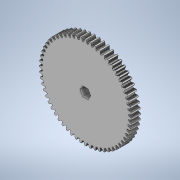
# Autodesk Inventor part: Engranajes_60
Saved by Autodesk Inventor 2022 (Build 260153000, 153)
## iProperties
Created: 2022-02-21
Part Number: Engranajes_60
Material: Generic
Document SubType Name: Modeling
Designer: katha
Density: 1 g/cm^3
Appearance: Default
Author: katha
Autodesk Inventor part; units mm, degrees
(part 1 of 6)
ref_plane "YZ Plane" through (0, 0, 0) normal (1, 0, 0) x (0, 1, 0)
ref_plane "XZ Plane" through (0, 0, 0) normal (0, 1, 0) x (-1, 0, 0)
ref_plane "XY Plane" through (0, 0, 0) normal (0, 0, 1) x (1, 0, 0)
sketch "Sketch1" plane through (0, 0, 0) normal (0, 0, 1) x (1, 0, 0)
  circle A0 centre (37.5, 0) radius 2
  circle A1 centre (0, 0) radius 2
  circle A2 centre (37.5, 0) radius 2
  circle A3 centre (0, 0) radius 2
  line L0 (30.5004, -4.5761) -> (30.5788, -4.4112)
  line L1 (30.5788, -4.4112) -> (30.6581, -4.2611)
  line L2 (30.6581, -4.2611) -> (30.7375, -4.1249)
  line L3 (30.7375, -4.1249) -> (30.8151, -4.0037)
  line L4 (30.8151, -4.0037) -> (30.8928, -3.8929)
  line L5 (30.8928, -3.8929) -> (30.9659, -3.7975)
  line L6 (30.9659, -3.7975) -> (31.0351, -3.7146)
  line L7 (31.0351, -3.7146) -> (31.0995, -3.6436)
  line L8 (31.0995, -3.6436) -> (31.1577, -3.5847)
  line L9 (31.1577, -3.5847) -> (31.2544, -3.498)
  line L10 (31.2544, -3.498) -> (31.3364, -3.4375)
  line L11 (31.3364, -3.4375) -> (31.3874, -3.4115)
  line L12 (31.3874, -3.4115) -> (31.4881, -3.3539)
  line L13 (31.4881, -3.3539) -> (31.5734, -3.2945)
  line L14 (31.5734, -3.2945) -> (31.6432, -3.2343)
  line L15 (31.6432, -3.2343) -> (31.6977, -3.1746)
  line L16 (31.6977, -3.1746) -> (31.7371, -3.1165)
  line L17 (31.7371, -3.1165) -> (31.7616, -3.0612)
  line L18 (31.7616, -3.0612) -> (31.7684, -3.035)
  line L19 (31.7684, -3.035) -> (31.7716, -3.0098)
  line L20 (31.7716, -3.0098) -> (31.7712, -2.986)
  line L21 (31.7712, -2.986) -> (31.7674, -2.9635)
  line L22 (31.7674, -2.9635) -> (31.7578, -2.9376)
  line L23 (31.7578, -2.9376) -> (31.6423, -2.7)
  line L24 (31.6423, -2.7) -> (31.6076, -2.6235)
  line L25 (31.6076, -2.6235) -> (31.5739, -2.5464)
  line L26 (31.5739, -2.5464) -> (31.4746, -2.3016)
  line L27 (31.4746, -2.3016) -> (31.4618, -2.2772)
  line L28 (31.4618, -2.2772) -> (31.4477, -2.2593)
  line L29 (31.4477, -2.2593) -> (31.4302, -2.2431)
  line L30 (31.4302, -2.2431) -> (31.4094, -2.2286)
  line L31 (31.4094, -2.2286) -> (31.3854, -2.2161)
  line L32 (31.3854, -2.2161) -> (31.3279, -2.1973)
  line L33 (31.3279, -2.1973) -> (31.2584, -2.1877)
  line L34 (31.2584, -2.1877) -> (31.1775, -2.1883)
  line L35 (31.1775, -2.1883) -> (31.0861, -2.1999)
  line L36 (31.0861, -2.1999) -> (30.9848, -2.2234)
  line L37 (30.9848, -2.2234) -> (30.8747, -2.2598)
  line L38 (30.8747, -2.2598) -> (30.8212, -2.2803)
  line L39 (30.8212, -2.2803) -> (30.7213, -2.3008)
  line L40 (30.7213, -2.3008) -> (30.5923, -2.3146)
  line L41 (30.5923, -2.3146) -> (30.5095, -2.3184)
  line L42 (30.5095, -2.3184) -> (30.4137, -2.3188)
  line L43 (30.4137, -2.3188) -> (30.3057, -2.3148)
  line L44 (30.3057, -2.3148) -> (30.186, -2.3053)
  line L45 (30.186, -2.3053) -> (30.0516, -2.2888)
  line L46 (30.0516, -2.2888) -> (29.9096, -2.2654)
  line L47 (29.9096, -2.2654) -> (29.7552, -2.2333)
  line L48 (29.7552, -2.2333) -> (29.5907, -2.1918)
  line L49 (29.5907, -2.1918) -> (29.4157, -2.1397)
  line L50 (29.4157, -2.1397) -> (29.2602, -2.0868)
  arc A4 (29.1238, -1.4451) -> (29.2602, -2.0868) centre (37.5, 0) ccw
  line L51 (29.1238, -1.4451) -> (29.2443, -1.3335)
  line L52 (29.2443, -1.3335) -> (29.383, -1.2147)
  line L53 (29.383, -1.2147) -> (29.5164, -1.1099)
  line L54 (29.5164, -1.1099) -> (29.6444, -1.0178)
  line L55 (29.6444, -1.0178) -> (29.7646, -0.9386)
  line L56 (29.7646, -0.9386) -> (29.8807, -0.8689)
  line L57 (29.8807, -0.8689) -> (29.9862, -0.8115)
  line L58 (29.9862, -0.8115) -> (30.0832, -0.7639)
  line L59 (30.0832, -0.7639) -> (30.1709, -0.7253)
  line L60 (30.1709, -0.7253) -> (30.248, -0.6951)
  line L61 (30.248, -0.6951) -> (30.3716, -0.6552)
  line L62 (30.3716, -0.6552) -> (30.4711, -0.6334)
  line L63 (30.4711, -0.6334) -> (30.5283, -0.6304)
  line L64 (30.5283, -0.6304) -> (30.6437, -0.6187)
  line L65 (30.6437, -0.6187) -> (30.7458, -0.5991)
  line L66 (30.7458, -0.5991) -> (30.8341, -0.5725)
  line L67 (30.8341, -0.5725) -> (30.9081, -0.5401)
  line L68 (30.9081, -0.5401) -> (30.9677, -0.5031)
  line L69 (30.9677, -0.5031) -> (31.0126, -0.4625)
  line L70 (31.0126, -0.4625) -> (31.0295, -0.4413)
  line L71 (31.0295, -0.4413) -> (31.0426, -0.4197)
  line L72 (31.0426, -0.4197) -> (31.052, -0.3977)
  line L73 (31.052, -0.3977) -> (31.0576, -0.3757)
  line L74 (31.0576, -0.3757) -> (31.0594, -0.3481)
  line L75 (31.0594, -0.3481) -> (31.0505, -0.0841)
  line L76 (31.0505, -0.0841) -> (31.05, 0)
  line L77 (31.05, 0) -> (31.0505, 0.0841)
  line L78 (31.0505, 0.0841) -> (31.0594, 0.3481)
  line L79 (31.0594, 0.3481) -> (31.0576, 0.3757)
  line L80 (31.0576, 0.3757) -> (31.052, 0.3977)
  line L81 (31.052, 0.3977) -> (31.0426, 0.4197)
  line L82 (31.0426, 0.4197) -> (31.0295, 0.4413)
  line L83 (31.0295, 0.4413) -> (31.0126, 0.4625)
  line L84 (31.0126, 0.4625) -> (30.9677, 0.5031)
  line L85 (30.9677, 0.5031) -> (30.9081, 0.5401)
  line L86 (30.9081, 0.5401) -> (30.8341, 0.5725)
  line L87 (30.8341, 0.5725) -> (30.7458, 0.5991)
  line L88 (30.7458, 0.5991) -> (30.6437, 0.6187)
  line L89 (30.6437, 0.6187) -> (30.5283, 0.6304)
  line L90 (30.5283, 0.6304) -> (30.4711, 0.6334)
  line L91 (30.4711, 0.6334) -> (30.3716, 0.6552)
  line L92 (30.3716, 0.6552) -> (30.248, 0.6951)
  line L93 (30.248, 0.6951) -> (30.1709, 0.7253)
  line L94 (30.1709, 0.7253) -> (30.0832, 0.7639)
  line L95 (30.0832, 0.7639) -> (29.9862, 0.8115)
  line L96 (29.9862, 0.8115) -> (29.8807, 0.8689)
  line L97 (29.8807, 0.8689) -> (29.7646, 0.9386)
  line L98 (29.7646, 0.9386) -> (29.6444, 1.0178)
  line L99 (29.6444, 1.0178) -> (29.5164, 1.1099)
  line L100 (29.5164, 1.1099) -> (29.383, 1.2147)
  line L101 (29.383, 1.2147) -> (29.2443, 1.3335)
  line L102 (29.2443, 1.3335) -> (29.1238, 1.4451)
  arc A5 (29.2602, 2.0868) -> (29.1238, 1.4451) centre (37.5, 0) ccw
  line L103 (29.2602, 2.0868) -> (29.4157, 2.1397)
  line L104 (29.4157, 2.1397) -> (29.5907, 2.1918)
  line L105 (29.5907, 2.1918) -> (29.7552, 2.2333)
  line L106 (29.7552, 2.2333) -> (29.9096, 2.2654)
  line L107 (29.9096, 2.2654) -> (30.0516, 2.2888)
  line L108 (30.0516, 2.2888) -> (30.186, 2.3053)
  line L109 (30.186, 2.3053) -> (30.3057, 2.3148)
  line L110 (30.3057, 2.3148) -> (30.4137, 2.3188)
  line L111 (30.4137, 2.3188) -> (30.5095, 2.3184)
  line L112 (30.5095, 2.3184) -> (30.5923, 2.3146)
  line L113 (30.5923, 2.3146) -> (30.7213, 2.3008)
  line L114 (30.7213, 2.3008) -> (30.8212, 2.2803)
  line L115 (30.8212, 2.2803) -> (30.8747, 2.2598)
  line L116 (30.8747, 2.2598) -> (30.9848, 2.2234)
  line L117 (30.9848, 2.2234) -> (31.0861, 2.1999)
  line L118 (31.0861, 2.1999) -> (31.1775, 2.1883)
  line L119 (31.1775, 2.1883) -> (31.2584, 2.1877)
  line L120 (31.2584, 2.1877) -> (31.3279, 2.1973)
  line L121 (31.3279, 2.1973) -> (31.3854, 2.2161)
  line L122 (31.3854, 2.2161) -> (31.4094, 2.2286)
  line L123 (31.4094, 2.2286) -> (31.4302, 2.2431)
  line L124 (31.4302, 2.2431) -> (31.4477, 2.2593)
  line L125 (31.4477, 2.2593) -> (31.4618, 2.2772)
  line L126 (31.4618, 2.2772) -> (31.4746, 2.3016)
  line L127 (31.4746, 2.3016) -> (31.5739, 2.5464)
  line L128 (31.5739, 2.5464) -> (31.6076, 2.6235)
  line L129 (31.6076, 2.6235) -> (31.6423, 2.7)
  line L130 (31.6423, 2.7) -> (31.7578, 2.9376)
  line L131 (31.7578, 2.9376) -> (31.7674, 2.9635)
  line L132 (31.7674, 2.9635) -> (31.7712, 2.986)
  line L133 (31.7712, 2.986) -> (31.7716, 3.0098)
  line L134 (31.7716, 3.0098) -> (31.7684, 3.035)
  line L135 (31.7684, 3.035) -> (31.7616, 3.0612)
  line L136 (31.7616, 3.0612) -> (31.7371, 3.1165)
  line L137 (31.7371, 3.1165) -> (31.6977, 3.1746)
  line L138 (31.6977, 3.1746) -> (31.6432, 3.2343)
  line L139 (31.6432, 3.2343) -> (31.5734, 3.2945)
  line L140 (31.5734, 3.2945) -> (31.4881, 3.3539)
  line L141 (31.4881, 3.3539) -> (31.3874, 3.4115)
  line L142 (31.3874, 3.4115) -> (31.3364, 3.4375)
  line L143 (31.3364, 3.4375) -> (31.2544, 3.498)
  line L144 (31.2544, 3.498) -> (31.1577, 3.5847)
  line L145 (31.1577, 3.5847) -> (31.0995, 3.6436)
  line L146 (31.0995, 3.6436) -> (31.0351, 3.7146)
  line L147 (31.0351, 3.7146) -> (30.9659, 3.7975)
  line L148 (30.9659, 3.7975) -> (30.8928, 3.8929)
  line L149 (30.8928, 3.8929) -> (30.8151, 4.0037)
  line L150 (30.8151, 4.0037) -> (30.7375, 4.1249)
  line L151 (30.7375, 4.1249) -> (30.6581, 4.2611)
  line L152 (30.6581, 4.2611) -> (30.5788, 4.4112)
  line L153 (30.5788, 4.4112) -> (30.5004, 4.5761)
  line L154 (30.5004, 4.5761) -> (30.4357, 4.7271)
  arc A6 (30.8213, 5.2578) -> (30.4357, 4.7271) centre (37.5, 0) ccw
  line L155 (30.8213, 5.2578) -> (30.9849, 5.243)
  line L156 (30.9849, 5.243) -> (31.1659, 5.2193)
  line L157 (31.1659, 5.2193) -> (31.3332, 5.1903)
  line L158 (31.3332, 5.1903) -> (31.4872, 5.1568)
  line L159 (31.4872, 5.1568) -> (31.6265, 5.1205)
  line L160 (31.6265, 5.1205) -> (31.756, 5.0808)
  line L161 (31.756, 5.0808) -> (31.8692, 5.0408)
  line L162 (31.8692, 5.0408) -> (31.9695, 5.0006)
  line L163 (31.9695, 5.0006) -> (32.0569, 4.9613)
  line L164 (32.0569, 4.9613) -> (32.1309, 4.9241)
  line L165 (32.1309, 4.9241) -> (32.2432, 4.859)
  line L166 (32.2432, 4.859) -> (32.3261, 4.7997)
  line L167 (32.3261, 4.7997) -> (32.3666, 4.7592)
  line L168 (32.3666, 4.7592) -> (32.4524, 4.6812)
  line L169 (32.4524, 4.6812) -> (32.5353, 4.6185)
  line L170 (32.5353, 4.6185) -> (32.6142, 4.5707)
  line L171 (32.6142, 4.5707) -> (32.6878, 4.5373)
  line L172 (32.6878, 4.5373) -> (32.7552, 4.5178)
  line L173 (32.7552, 4.5178) -> (32.8154, 4.5116)
  line L174 (32.8154, 4.5116) -> (32.8424, 4.5132)
  line L175 (32.8424, 4.5132) -> (32.8673, 4.518)
  line L176 (32.8673, 4.518) -> (32.8899, 4.5257)
  line L177 (32.8899, 4.5257) -> (32.9101, 4.5363)
  line L178 (32.9101, 4.5363) -> (32.9317, 4.5534)
  line L179 (32.9317, 4.5534) -> (33.122, 4.7366)
  line L180 (33.122, 4.7366) -> (33.1841, 4.7933)
  line L181 (33.1841, 4.7933) -> (33.2469, 4.8492)
  line L182 (33.2469, 4.8492) -> (33.4491, 5.0192)
  line L183 (33.4491, 5.0192) -> (33.4684, 5.039)
  line L184 (33.4684, 5.039) -> (33.481, 5.0579)
  line L185 (33.481, 5.0579) -> (33.491, 5.0796)
  line L186 (33.491, 5.0796) -> (33.4983, 5.1038)
  line L187 (33.4983, 5.1038) -> (33.5028, 5.1306)
  line L188 (33.5028, 5.1306) -> (33.5029, 5.191)
  line L189 (33.5029, 5.191) -> (33.4906, 5.2601)
  line L190 (33.4906, 5.2601) -> (33.4651, 5.3368)
  line L191 (33.4651, 5.3368) -> (33.4258, 5.4202)
  line L192 (33.4258, 5.4202) -> (33.3721, 5.5092)
  line L193 (33.3721, 5.5092) -> (33.3035, 5.6028)
  line L194 (33.3035, 5.6028) -> (33.2674, 5.6473)
  line L195 (33.2674, 5.6473) -> (33.2171, 5.7359)
  line L196 (33.2171, 5.7359) -> (33.1641, 5.8544)
  line L197 (33.1641, 5.8544) -> (33.1349, 5.9319)
  line L198 (33.1349, 5.9319) -> (33.1049, 6.0229)
  line L199 (33.1049, 6.0229) -> (33.0754, 6.1269)
  line L200 (33.0754, 6.1269) -> (33.0474, 6.2437)
  line L201 (33.0474, 6.2437) -> (33.0215, 6.3765)
  line L202 (33.0215, 6.3765) -> (32.9999, 6.5189)
  line L203 (32.9999, 6.5189) -> (32.9828, 6.6756)
  line L204 (32.9828, 6.6756) -> (32.9714, 6.8449)
  line L205 (32.9714, 6.8449) -> (32.9668, 7.0275)
  line L206 (32.9668, 7.0275) -> (32.9691, 7.1917)
  arc A7 (33.5372, 7.5197) -> (32.9691, 7.1917) centre (37.5, 0) ccw
  line L207 (33.5372, 7.5197) -> (33.6807, 7.4396)
  line L208 (33.6807, 7.4396) -> (33.8364, 7.3444)
  line L209 (33.8364, 7.3444) -> (33.9774, 7.2498)
  line L210 (33.9774, 7.2498) -> (34.1045, 7.1566)
  line L211 (34.1045, 7.1566) -> (34.217, 7.0668)
  line L212 (34.217, 7.0668) -> (34.3191, 6.9779)
  line L213 (34.3191, 6.9779) -> (34.4063, 6.8953)
  line L214 (34.4063, 6.8953) -> (34.4815, 6.8178)
  line L215 (34.4815, 6.8178) -> (34.5454, 6.7463)
  line L216 (34.5454, 6.7463) -> (34.5979, 6.6822)
  line L217 (34.5979, 6.6822) -> (34.674, 6.5771)
  line L218 (34.674, 6.5771) -> (34.7256, 6.4892)
  line L219 (34.7256, 6.4892) -> (34.7461, 6.4357)
  line L220 (34.7461, 6.4357) -> (34.7928, 6.3295)
  line L221 (34.7928, 6.3295) -> (34.8431, 6.2385)
  line L222 (34.8431, 6.2385) -> (34.8956, 6.1628)
  line L223 (34.8956, 6.1628) -> (34.9493, 6.1023)
  line L224 (34.9493, 6.1023) -> (35.003, 6.0571)
  line L225 (35.003, 6.0571) -> (35.0554, 6.0269)
  line L226 (35.0554, 6.0269) -> (35.0808, 6.0175)
  line L227 (35.0808, 6.0175) -> (35.1054, 6.0117)
  line L228 (35.1054, 6.0117) -> (35.1292, 6.0095)
  line L229 (35.1292, 6.0095) -> (35.1519, 6.011)
  line L230 (35.1519, 6.011) -> (35.1787, 6.0178)
  line L231 (35.1787, 6.0178) -> (35.427, 6.1078)
  line L232 (35.427, 6.1078) -> (35.5068, 6.1343)
  line L233 (35.5068, 6.1343) -> (35.587, 6.1598)
  line L234 (35.587, 6.1598) -> (35.8408, 6.2329)
  line L235 (35.8408, 6.2329) -> (35.8665, 6.2431)
  line L236 (35.8665, 6.2431) -> (35.8857, 6.2553)
  line L237 (35.8857, 6.2553) -> (35.9037, 6.271)
  line L238 (35.9037, 6.271) -> (35.9202, 6.2902)
  line L239 (35.9202, 6.2902) -> (35.9352, 6.3128)
  line L240 (35.9352, 6.3128) -> (35.9599, 6.368)
  line L241 (35.9599, 6.368) -> (35.9767, 6.4361)
  line L242 (35.9767, 6.4361) -> (35.9846, 6.5166)
  line L243 (35.9846, 6.5166) -> (35.9826, 6.6088)
  line L244 (35.9826, 6.6088) -> (35.9698, 6.7119)
  line L245 (35.9698, 6.7119) -> (35.9451, 6.8253)
  line L246 (35.9451, 6.8253) -> (35.9303, 6.8806)
  line L247 (35.9303, 6.8806) -> (35.9204, 6.982)
  line L248 (35.9204, 6.982) -> (35.9201, 7.1118)
  line L249 (35.9201, 7.1118) -> (35.925, 7.1945)
  line L250 (35.925, 7.1945) -> (35.9346, 7.2899)
  line L251 (35.9346, 7.2899) -> (35.9499, 7.3968)
  line L252 (35.9499, 7.3968) -> (35.9719, 7.5149)
  line L253 (35.9719, 7.5149) -> (36.0023, 7.6468)
  line L254 (36.0023, 7.6468) -> (36.0404, 7.7856)
  line L255 (36.0404, 7.7856) -> (36.0885, 7.9358)
  line L256 (36.0885, 7.9358) -> (36.147, 8.0951)
  line L257 (36.147, 8.0951) -> (36.217, 8.2637)
  line L258 (36.217, 8.2637) -> (36.286, 8.4128)
  arc A8 (36.9384, 8.4814) -> (36.286, 8.4128) centre (37.5, 0) ccw
  line L259 (36.9384, 8.4814) -> (37.0368, 8.3499)
  line L260 (37.0368, 8.3499) -> (37.1404, 8.1995)
  line L261 (37.1404, 8.1995) -> (37.2307, 8.0558)
  line L262 (37.2307, 8.0558) -> (37.309, 7.919)
  line L263 (37.309, 7.919) -> (37.3751, 7.7911)
  line L264 (37.3751, 7.7911) -> (37.4323, 7.6684)
  line L265 (37.4323, 7.6684) -> (37.4783, 7.5575)
  line L266 (37.4783, 7.5575) -> (37.5155, 7.4561)
  line L267 (37.5155, 7.4561) -> (37.5448, 7.3648)
  line L268 (37.5448, 7.3648) -> (37.5667, 7.2849)
  line L269 (37.5667, 7.2849) -> (37.5935, 7.1579)
  line L270 (37.5935, 7.1579) -> (37.6048, 7.0566)
  line L271 (37.6048, 7.0566) -> (37.6018, 6.9994)
  line L272 (37.6018, 6.9994) -> (37.6013, 6.8834)
  line L273 (37.6013, 6.8834) -> (37.6102, 6.7798)
  line L274 (37.6102, 6.7798) -> (37.6274, 6.6893)
  line L275 (37.6274, 6.6893) -> (37.6519, 6.6122)
  line L276 (37.6519, 6.6122) -> (37.6825, 6.5491)
  line L277 (37.6825, 6.5491) -> (37.7181, 6.5002)
  line L278 (37.7181, 6.5002) -> (37.7375, 6.4812)
  line L279 (37.7375, 6.4812) -> (37.7576, 6.4659)
  line L280 (37.7576, 6.4659) -> (37.7784, 6.4543)
  line L281 (37.7784, 6.4543) -> (37.7998, 6.4463)
  line L282 (37.7998, 6.4463) -> (37.8271, 6.4417)
  line L283 (37.8271, 6.4417) -> (38.0905, 6.4229)
  line L284 (38.0905, 6.4229) -> (38.1742, 6.4147)
  line L285 (38.1742, 6.4147) -> (38.2578, 6.4054)
  line L286 (38.2578, 6.4054) -> (38.5194, 6.3689)
  line L287 (38.5194, 6.3689) -> (38.547, 6.3678)
  line L288 (38.547, 6.3678) -> (38.5696, 6.3711)
  line L289 (38.5696, 6.3711) -> (38.5923, 6.3781)
  line L290 (38.5923, 6.3781) -> (38.6152, 6.3889)
  line L291 (38.6152, 6.3889) -> (38.6381, 6.4035)
  line L292 (38.6381, 6.4035) -> (38.6831, 6.4439)
  line L293 (38.6831, 6.4439) -> (38.7262, 6.4993)
  line L294 (38.7262, 6.4993) -> (38.7661, 6.5696)
  line L295 (38.7661, 6.5696) -> (38.8018, 6.6546)
  line L296 (38.8018, 6.6546) -> (38.832, 6.754)
  line L297 (38.832, 6.754) -> (38.8557, 6.8676)
  line L298 (38.8557, 6.8676) -> (38.8646, 6.9242)
  line L299 (38.8646, 6.9242) -> (38.8968, 7.0209)
  line L300 (38.8968, 7.0209) -> (38.9493, 7.1396)
  line L301 (38.9493, 7.1396) -> (38.9874, 7.2131)
  line L302 (38.9874, 7.2131) -> (39.035, 7.2964)
  line L303 (39.035, 7.2964) -> (39.0925, 7.3878)
  line L304 (39.0925, 7.3878) -> (39.1606, 7.4867)
  line L305 (39.1606, 7.4867) -> (39.242, 7.5949)
  line L306 (39.242, 7.5949) -> (39.3333, 7.7062)
  line L307 (39.3333, 7.7062) -> (39.4383, 7.8238)
  line L308 (39.4383, 7.8238) -> (39.5565, 7.9456)
  line L309 (39.5565, 7.9456) -> (39.6891, 8.0711)
  line L310 (39.6891, 8.0711) -> (39.8127, 8.1793)
  arc A9 (40.4366, 7.9766) -> (39.8127, 8.1793) centre (37.5, 0) ccw
  line L311 (40.4366, 7.9766) -> (40.4731, 7.8164)
  line L312 (40.4731, 7.8164) -> (40.5065, 7.6369)
  line L313 (40.5065, 7.6369) -> (40.5306, 7.4689)
  line L314 (40.5306, 7.4689) -> (40.5464, 7.312)
  line L315 (40.5464, 7.312) -> (40.5549, 7.1683)
  line L316 (40.5549, 7.1683) -> (40.5571, 7.033)
  line L317 (40.5571, 7.033) -> (40.5541, 6.9129)
  line L318 (40.5541, 6.9129) -> (40.5468, 6.8051)
  line L319 (40.5468, 6.8051) -> (40.5364, 6.7098)
  line L320 (40.5364, 6.7098) -> (40.524, 6.628)
  line L321 (40.524, 6.628) -> (40.4968, 6.501)
  line L322 (40.4968, 6.501) -> (40.466, 6.4039)
  line L323 (40.466, 6.4039) -> (40.4399, 6.3528)
  line L324 (40.4399, 6.3528) -> (40.3923, 6.2471)
  line L325 (40.3923, 6.2471) -> (40.3583, 6.1489)
  line L326 (40.3583, 6.1489) -> (40.3372, 6.0591)
  line L327 (40.3372, 6.0591) -> (40.3282, 5.9788)
  line L328 (40.3282, 5.9788) -> (40.3305, 5.9086)
  line L329 (40.3305, 5.9086) -> (40.3431, 5.8495)
  line L330 (40.3431, 5.8495) -> (40.3531, 5.8243)
  line L331 (40.3531, 5.8243) -> (40.3653, 5.8021)
  line L332 (40.3653, 5.8021) -> (40.3796, 5.783)
  line L333 (40.3796, 5.783) -> (40.3959, 5.7671)
  line L334 (40.3959, 5.7671) -> (40.4189, 5.7518)
  line L335 (40.4189, 5.7518) -> (40.6519, 5.6274)
  line L336 (40.6519, 5.6274) -> (40.725, 5.5859)
  line L337 (40.725, 5.5859) -> (40.7976, 5.5434)
  line L338 (40.7976, 5.5434) -> (41.0218, 5.4037)
  line L339 (41.0218, 5.4037) -> (41.0465, 5.3914)
  line L340 (41.0465, 5.3914) -> (41.0684, 5.3853)
  line L341 (41.0684, 5.3853) -> (41.0921, 5.3824)
  line L342 (41.0921, 5.3824) -> (41.1174, 5.383)
  line L343 (41.1174, 5.383) -> (41.1443, 5.387)
  line L344 (41.1443, 5.387) -> (41.2018, 5.4056)
  line L345 (41.2018, 5.4056) -> (41.2637, 5.4387)
  line L346 (41.2637, 5.4387) -> (41.3288, 5.4866)
  line L347 (41.3288, 5.4866) -> (41.3959, 5.5498)
  line L348 (41.3959, 5.5498) -> (41.464, 5.6283)
  line L349 (41.464, 5.6283) -> (41.5318, 5.7225)
  line L350 (41.5318, 5.7225) -> (41.563, 5.7705)
  line L351 (41.563, 5.7705) -> (41.6317, 5.8458)
  line L352 (41.6317, 5.8458) -> (41.728, 5.9328)
  line L353 (41.728, 5.9328) -> (41.7927, 5.9845)
  line L354 (41.7927, 5.9845) -> (41.87, 6.0412)
  line L355 (41.87, 6.0412) -> (41.9597, 6.1014)
  line L356 (41.9597, 6.1014) -> (42.0622, 6.1641)
  line L357 (42.0622, 6.1641) -> (42.1805, 6.2298)
  line L358 (42.1805, 6.2298) -> (42.3092, 6.2943)
  line L359 (42.3092, 6.2943) -> (42.453, 6.359)
  line L360 (42.453, 6.359) -> (42.6105, 6.4222)
  line L361 (42.6105, 6.4222) -> (42.7827, 6.4829)
  line L362 (42.7827, 6.4829) -> (42.9396, 6.5315)
  arc A10 (43.4271, 6.0925) -> (42.9396, 6.5315) centre (37.5, 0) ccw
  line L363 (43.4271, 6.0925) -> (43.3952, 5.9314)
  line L364 (43.3952, 5.9314) -> (43.3528, 5.7538)
  line L365 (43.3528, 5.7538) -> (43.3065, 5.5905)
  line L366 (43.3065, 5.5905) -> (43.2571, 5.4408)
  line L367 (43.2571, 5.4408) -> (43.2064, 5.3061)
  line L368 (43.2064, 5.3061) -> (43.1534, 5.1815)
  line L369 (43.1534, 5.1815) -> (43.1018, 5.073)
  line L370 (43.1018, 5.073) -> (43.0513, 4.9775)
  line L371 (43.0513, 4.9775) -> (43.003, 4.8947)
  line L372 (43.003, 4.8947) -> (42.9584, 4.825)
  line L373 (42.9584, 4.825) -> (42.8819, 4.7201)
  line L374 (42.8819, 4.7201) -> (42.8142, 4.6439)
  line L375 (42.8142, 4.6439) -> (42.7697, 4.6078)
  line L376 (42.7697, 4.6078) -> (42.6832, 4.5306)
  line L377 (42.6832, 4.5306) -> (42.6121, 4.4547)
  line L378 (42.6121, 4.4547) -> (42.5564, 4.3813)
  line L379 (42.5564, 4.3813) -> (42.5155, 4.3115)
  line L380 (42.5155, 4.3115) -> (42.489, 4.2466)
  line L381 (42.489, 4.2466) -> (42.4765, 4.1874)
  line L382 (42.4765, 4.1874) -> (42.4754, 4.1603)
  line L383 (42.4754, 4.1603) -> (42.4775, 4.1351)
  line L384 (42.4775, 4.1351) -> (42.4828, 4.1118)
  line L385 (42.4828, 4.1118) -> (42.4912, 4.0906)
  line L386 (42.4912, 4.0906) -> (42.506, 4.0673)
  line L387 (42.506, 4.0673) -> (42.6683, 3.8589)
  line L388 (42.6683, 3.8589) -> (42.7182, 3.7912)
  line L389 (42.7182, 3.7912) -> (42.7672, 3.7229)
  line L390 (42.7672, 3.7229) -> (42.9152, 3.5041)
  line L391 (42.9152, 3.5041) -> (42.9328, 3.4828)
  line L392 (42.9328, 3.4828) -> (42.9503, 3.4683)
  line L393 (42.9503, 3.4683) -> (42.9708, 3.456)
  line L394 (42.9708, 3.456) -> (42.9942, 3.4462)
  line L395 (42.9942, 3.4462) -> (43.0203, 3.439)
  line L396 (43.0203, 3.439) -> (43.0804, 3.4326)
  line L397 (43.0804, 3.4326) -> (43.1504, 3.4376)
  line L398 (43.1504, 3.4376) -> (43.2294, 3.455)
  line L399 (43.2294, 3.455) -> (43.3164, 3.4854)
  line L400 (43.3164, 3.4854) -> (43.4105, 3.5294)
  line L401 (43.4105, 3.5294) -> (43.5107, 3.5879)
  line L402 (43.5107, 3.5879) -> (43.5588, 3.6191)
  line L403 (43.5588, 3.6191) -> (43.6522, 3.6599)
  line L404 (43.6522, 3.6599) -> (43.7755, 3.7002)
  line L405 (43.7755, 3.7002) -> (43.8557, 3.7212)
  line L406 (43.8557, 3.7212) -> (43.9494, 3.7415)
  line L407 (43.9494, 3.7415) -> (44.0558, 3.76)
  line L408 (44.0558, 3.76) -> (44.1749, 3.7755)
  line L409 (44.1749, 3.7755) -> (44.3097, 3.7874)
  line L410 (44.3097, 3.7874) -> (44.4536, 3.794)
  line L411 (44.4536, 3.794) -> (44.6112, 3.7947)
  line L412 (44.6112, 3.7947) -> (44.7808, 3.7883)
  line L413 (44.7808, 3.7883) -> (44.9628, 3.7738)
  line L414 (44.9628, 3.7738) -> (45.1259, 3.7543)
  arc A11 (45.3927, 3.155) -> (45.1259, 3.7543) centre (37.5, 0) ccw
  line L415 (45.3927, 3.155) -> (45.2981, 3.0208)
  line L416 (45.2981, 3.0208) -> (45.1871, 2.8758)
  line L417 (45.1871, 2.8758) -> (45.0783, 2.7455)
  line L418 (45.0783, 2.7455) -> (44.9724, 2.6288)
  line L419 (44.9724, 2.6288) -> (44.8712, 2.5263)
  line L420 (44.8712, 2.5263) -> (44.7722, 2.4341)
  line L421 (44.7722, 2.4341) -> (44.6809, 2.356)
  line L422 (44.6809, 2.356) -> (44.5959, 2.2893)
  line L423 (44.5959, 2.2893) -> (44.5181, 2.2332)
  line L424 (44.5181, 2.2332) -> (44.449, 2.1877)
  line L425 (44.449, 2.1877) -> (44.3364, 2.123)
  line L426 (44.3364, 2.123) -> (44.2436, 2.0809)
  line L427 (44.2436, 2.0809) -> (44.1883, 2.0661)
  line L428 (44.1883, 2.0661) -> (44.0778, 2.0307)
  line L429 (44.0778, 2.0307) -> (43.9821, 1.9903)
  line L430 (43.9821, 1.9903) -> (43.9013, 1.9459)
  line L431 (43.9013, 1.9459) -> (43.8355, 1.8988)
  line L432 (43.8355, 1.8988) -> (43.7849, 1.8502)
  line L433 (43.7849, 1.8502) -> (43.7494, 1.8012)
  line L434 (43.7494, 1.8012) -> (43.7374, 1.777)
  line L435 (43.7374, 1.777) -> (43.729, 1.7531)
  line L436 (43.729, 1.7531) -> (43.7244, 1.7297)
  line L437 (43.7244, 1.7297) -> (43.7235, 1.7069)
  line L438 (43.7235, 1.7069) -> (43.7275, 1.6796)
  line L439 (43.7275, 1.6796) -> (43.7911, 1.4232)
  line L440 (43.7911, 1.4232) -> (43.8091, 1.341)
  line L441 (43.8091, 1.341) -> (43.826, 1.2587)
  line L442 (43.826, 1.2587) -> (43.8722, 0.9986)
  line L443 (43.8722, 0.9986) -> (43.8797, 0.972)
  line L444 (43.8797, 0.972) -> (43.8898, 0.9516)
  line L445 (43.8898, 0.9516) -> (43.9035, 0.9321)
  line L446 (43.9035, 0.9321) -> (43.9209, 0.9136)
  line L447 (43.9209, 0.9136) -> (43.9418, 0.8964)
  line L448 (43.9418, 0.8964) -> (43.9941, 0.8661)
  line L449 (43.9941, 0.8661) -> (44.0601, 0.8422)
  line L450 (44.0601, 0.8422) -> (44.1393, 0.8259)
  line L451 (44.1393, 0.8259) -> (44.2312, 0.8183)
  line L452 (44.2312, 0.8183) -> (44.3351, 0.8203)
  line L453 (44.3351, 0.8203) -> (44.4504, 0.8329)
  line L454 (44.4504, 0.8329) -> (44.507, 0.8419)
  line L455 (44.507, 0.8419) -> (44.6089, 0.8412)
  line L456 (44.6089, 0.8412) -> (44.738, 0.8278)
  line L457 (44.738, 0.8278) -> (44.8197, 0.8144)
  line L458 (44.8197, 0.8144) -> (44.9136, 0.7948)
  line L459 (44.9136, 0.7948) -> (45.0183, 0.7684)
  line L460 (45.0183, 0.7684) -> (45.1335, 0.7342)
  line L461 (45.1335, 0.7342) -> (45.2615, 0.6902)
  line L462 (45.2615, 0.6902) -> (45.3956, 0.6378)
  line L463 (45.3956, 0.6378) -> (45.5398, 0.5742)
  line L464 (45.5398, 0.5742) -> (45.6922, 0.4994)
  line L465 (45.6922, 0.4994) -> (45.8526, 0.4122)
  line L466 (45.8526, 0.4122) -> (45.9936, 0.328)
  arc A12 (45.9936, -0.328) -> (45.9936, 0.328) centre (37.5, 0) ccw
  line L467 (45.9936, -0.328) -> (45.8526, -0.4122)
  line L468 (45.8526, -0.4122) -> (45.6922, -0.4994)
  line L469 (45.6922, -0.4994) -> (45.5398, -0.5742)
  line L470 (45.5398, -0.5742) -> (45.3956, -0.6378)
  line L471 (45.3956, -0.6378) -> (45.2615, -0.6902)
  line L472 (45.2615, -0.6902) -> (45.1335, -0.7342)
  line L473 (45.1335, -0.7342) -> (45.0183, -0.7684)
  line L474 (45.0183, -0.7684) -> (44.9136, -0.7948)
  line L475 (44.9136, -0.7948) -> (44.8197, -0.8144)
  line L476 (44.8197, -0.8144) -> (44.738, -0.8278)
  line L477 (44.738, -0.8278) -> (44.6089, -0.8412)
  line L478 (44.6089, -0.8412) -> (44.507, -0.8419)
  line L479 (44.507, -0.8419) -> (44.4504, -0.8329)
  line L480 (44.4504, -0.8329) -> (44.3351, -0.8203)
  line L481 (44.3351, -0.8203) -> (44.2312, -0.8183)
  line L482 (44.2312, -0.8183) -> (44.1393, -0.8259)
  line L483 (44.1393, -0.8259) -> (44.0601, -0.8422)
  line L484 (44.0601, -0.8422) -> (43.9941, -0.8661)
  line L485 (43.9941, -0.8661) -> (43.9418, -0.8964)
  line L486 (43.9418, -0.8964) -> (43.9209, -0.9136)
  line L487 (43.9209, -0.9136) -> (43.9035, -0.9321)
  line L488 (43.9035, -0.9321) -> (43.8898, -0.9516)
  line L489 (43.8898, -0.9516) -> (43.8797, -0.972)
  line L490 (43.8797, -0.972) -> (43.8722, -0.9986)
  line L491 (43.8722, -0.9986) -> (43.826, -1.2587)
  line L492 (43.826, -1.2587) -> (43.8091, -1.341)
  line L493 (43.8091, -1.341) -> (43.7911, -1.4232)
  line L494 (43.7911, -1.4232) -> (43.7275, -1.6796)
  line L495 (43.7275, -1.6796) -> (43.7235, -1.7069)
  line L496 (43.7235, -1.7069) -> (43.7244, -1.7297)
  line L497 (43.7244, -1.7297) -> (43.729, -1.7531)
  line L498 (43.729, -1.7531) -> (43.7374, -1.777)
  line L499 (43.7374, -1.777) -> (43.7494, -1.8012)
  line L500 (43.7494, -1.8012) -> (43.7849, -1.8502)
  line L501 (43.7849, -1.8502) -> (43.8355, -1.8988)
  line L502 (43.8355, -1.8988) -> (43.9013, -1.9459)
  line L503 (43.9013, -1.9459) -> (43.9821, -1.9903)
  line L504 (43.9821, -1.9903) -> (44.0778, -2.0307)
  line L505 (44.0778, -2.0307) -> (44.1883, -2.0661)
  line L506 (44.1883, -2.0661) -> (44.2436, -2.0809)
  line L507 (44.2436, -2.0809) -> (44.3364, -2.123)
  line L508 (44.3364, -2.123) -> (44.449, -2.1877)
  line L509 (44.449, -2.1877) -> (44.5181, -2.2332)
  line L510 (44.5181, -2.2332) -> (44.5959, -2.2893)
  line L511 (44.5959, -2.2893) -> (44.6809, -2.356)
  line L512 (44.6809, -2.356) -> (44.7722, -2.4341)
  line L513 (44.7722, -2.4341) -> (44.8712, -2.5263)
  line L514 (44.8712, -2.5263) -> (44.9724, -2.6288)
  line L515 (44.9724, -2.6288) -> (45.0783, -2.7455)
  line L516 (45.0783, -2.7455) -> (45.1871, -2.8758)
  line L517 (45.1871, -2.8758) -> (45.2981, -3.0208)
  line L518 (45.2981, -3.0208) -> (45.3927, -3.155)
  arc A13 (45.1259, -3.7543) -> (45.3927, -3.155) centre (37.5, 0) ccw
  line L519 (45.1259, -3.7543) -> (44.9628, -3.7738)
  line L520 (44.9628, -3.7738) -> (44.7808, -3.7883)
  line L521 (44.7808, -3.7883) -> (44.6112, -3.7947)
  line L522 (44.6112, -3.7947) -> (44.4536, -3.794)
  line L523 (44.4536, -3.794) -> (44.3097, -3.7874)
  line L524 (44.3097, -3.7874) -> (44.1749, -3.7755)
  line L525 (44.1749, -3.7755) -> (44.0558, -3.76)
  line L526 (44.0558, -3.76) -> (43.9494, -3.7415)
  line L527 (43.9494, -3.7415) -> (43.8557, -3.7212)
  line L528 (43.8557, -3.7212) -> (43.7755, -3.7002)
  line L529 (43.7755, -3.7002) -> (43.6522, -3.6599)
  line L530 (43.6522, -3.6599) -> (43.5588, -3.6191)
  line L531 (43.5588, -3.6191) -> (43.5107, -3.5879)
  line L532 (43.5107, -3.5879) -> (43.4105, -3.5294)
  line L533 (43.4105, -3.5294) -> (43.3164, -3.4854)
  line L534 (43.3164, -3.4854) -> (43.2294, -3.455)
  line L535 (43.2294, -3.455) -> (43.1504, -3.4376)
  line L536 (43.1504, -3.4376) -> (43.0804, -3.4326)
  line L537 (43.0804, -3.4326) -> (43.0203, -3.439)
  line L538 (43.0203, -3.439) -> (42.9942, -3.4462)
  line L539 (42.9942, -3.4462) -> (42.9708, -3.456)
  line L540 (42.9708, -3.456) -> (42.9503, -3.4683)
  line L541 (42.9503, -3.4683) -> (42.9328, -3.4828)
  line L542 (42.9328, -3.4828) -> (42.9152, -3.5041)
  line L543 (42.9152, -3.5041) -> (42.7672, -3.7229)
  line L544 (42.7672, -3.7229) -> (42.7182, -3.7912)
  line L545 (42.7182, -3.7912) -> (42.6683, -3.8589)
  line L546 (42.6683, -3.8589) -> (42.506, -4.0673)
  line L547 (42.506, -4.0673) -> (42.4912, -4.0906)
  line L548 (42.4912, -4.0906) -> (42.4828, -4.1118)
  line L549 (42.4828, -4.1118) -> (42.4775, -4.1351)
  line L550 (42.4775, -4.1351) -> (42.4754, -4.1603)
  line L551 (42.4754, -4.1603) -> (42.4765, -4.1874)
  line L552 (42.4765, -4.1874) -> (42.489, -4.2466)
  line L553 (42.489, -4.2466) -> (42.5155, -4.3115)
  line L554 (42.5155, -4.3115) -> (42.5564, -4.3813)
  line L555 (42.5564, -4.3813) -> (42.6121, -4.4547)
  line L556 (42.6121, -4.4547) -> (42.6832, -4.5306)
  line L557 (42.6832, -4.5306) -> (42.7697, -4.6078)
  line L558 (42.7697, -4.6078) -> (42.8142, -4.6439)
  line L559 (42.8142, -4.6439) -> (42.8819, -4.7201)
  line L560 (42.8819, -4.7201) -> (42.9584, -4.825)
  line L561 (42.9584, -4.825) -> (43.003, -4.8947)
  line L562 (43.003, -4.8947) -> (43.0513, -4.9775)
  line L563 (43.0513, -4.9775) -> (43.1018, -5.073)
  line L564 (43.1018, -5.073) -> (43.1534, -5.1815)
  line L565 (43.1534, -5.1815) -> (43.2064, -5.3061)
  line L566 (43.2064, -5.3061) -> (43.2571, -5.4408)
  line L567 (43.2571, -5.4408) -> (43.3065, -5.5905)
  line L568 (43.3065, -5.5905) -> (43.3528, -5.7538)
  line L569 (43.3528, -5.7538) -> (43.3952, -5.9314)
  line L570 (43.3952, -5.9314) -> (43.4271, -6.0925)
  arc A14 (42.9396, -6.5315) -> (43.4271, -6.0925) centre (37.5, 0) ccw
  line L571 (42.9396, -6.5315) -> (42.7827, -6.4829)
  line L572 (42.7827, -6.4829) -> (42.6105, -6.4222)
  line L573 (42.6105, -6.4222) -> (42.453, -6.359)
  line L574 (42.453, -6.359) -> (42.3092, -6.2943)
  line L575 (42.3092, -6.2943) -> (42.1805, -6.2298)
  line L576 (42.1805, -6.2298) -> (42.0622, -6.1641)
  line L577 (42.0622, -6.1641) -> (41.9597, -6.1014)
  line L578 (41.9597, -6.1014) -> (41.87, -6.0412)
  line L579 (41.87, -6.0412) -> (41.7927, -5.9845)
  line L580 (41.7927, -5.9845) -> (41.728, -5.9328)
  line L581 (41.728, -5.9328) -> (41.6317, -5.8458)
  line L582 (41.6317, -5.8458) -> (41.563, -5.7705)
  line L583 (41.563, -5.7705) -> (41.5318, -5.7225)
  line L584 (41.5318, -5.7225) -> (41.464, -5.6283)
  line L585 (41.464, -5.6283) -> (41.3959, -5.5498)
  line L586 (41.3959, -5.5498) -> (41.3288, -5.4866)
  line L587 (41.3288, -5.4866) -> (41.2637, -5.4387)
  line L588 (41.2637, -5.4387) -> (41.2018, -5.4056)
  line L589 (41.2018, -5.4056) -> (41.1443, -5.387)
  line L590 (41.1443, -5.387) -> (41.1174, -5.383)
  line L591 (41.1174, -5.383) -> (41.0921, -5.3824)
  line L592 (41.0921, -5.3824) -> (41.0684, -5.3853)
  line L593 (41.0684, -5.3853) -> (41.0465, -5.3914)
  line L594 (41.0465, -5.3914) -> (41.0218, -5.4037)
  line L595 (41.0218, -5.4037) -> (40.7976, -5.5434)
  line L596 (40.7976, -5.5434) -> (40.725, -5.5859)
  line L597 (40.725, -5.5859) -> (40.6519, -5.6274)
  line L598 (40.6519, -5.6274) -> (40.4189, -5.7518)
  line L599 (40.4189, -5.7518) -> (40.3959, -5.7671)
  line L600 (40.3959, -5.7671) -> (40.3796, -5.783)
  line L601 (40.3796, -5.783) -> (40.3653, -5.8021)
  line L602 (40.3653, -5.8021) -> (40.3531, -5.8243)
  line L603 (40.3531, -5.8243) -> (40.3431, -5.8495)
  line L604 (40.3431, -5.8495) -> (40.3305, -5.9086)
  line L605 (40.3305, -5.9086) -> (40.3282, -5.9788)
  line L606 (40.3282, -5.9788) -> (40.3372, -6.0591)
  line L607 (40.3372, -6.0591) -> (40.3583, -6.1489)
  line L608 (40.3583, -6.1489) -> (40.3923, -6.2471)
  line L609 (40.3923, -6.2471) -> (40.4399, -6.3528)
  line L610 (40.4399, -6.3528) -> (40.466, -6.4039)
  line L611 (40.466, -6.4039) -> (40.4968, -6.501)
  line L612 (40.4968, -6.501) -> (40.524, -6.628)
  line L613 (40.524, -6.628) -> (40.5364, -6.7098)
  line L614 (40.5364, -6.7098) -> (40.5468, -6.8051)
  line L615 (40.5468, -6.8051) -> (40.5541, -6.9129)
  line L616 (40.5541, -6.9129) -> (40.5571, -7.033)
  line L617 (40.5571, -7.033) -> (40.5549, -7.1683)
  line L618 (40.5549, -7.1683) -> (40.5464, -7.312)
  line L619 (40.5464, -7.312) -> (40.5306, -7.4689)
  line L620 (40.5306, -7.4689) -> (40.5065, -7.6369)
  line L621 (40.5065, -7.6369) -> (40.4731, -7.8164)
  line L622 (40.4731, -7.8164) -> (40.4366, -7.9766)
  arc A15 (39.8127, -8.1793) -> (40.4366, -7.9766) centre (37.5, 0) ccw
  line L623 (39.8127, -8.1793) -> (39.6891, -8.0711)
  line L624 (39.6891, -8.0711) -> (39.5565, -7.9456)
  line L625 (39.5565, -7.9456) -> (39.4383, -7.8238)
  line L626 (39.4383, -7.8238) -> (39.3333, -7.7062)
  line L627 (39.3333, -7.7062) -> (39.242, -7.5949)
  line L628 (39.242, -7.5949) -> (39.1606, -7.4867)
  line L629 (39.1606, -7.4867) -> (39.0925, -7.3878)
  line L630 (39.0925, -7.3878) -> (39.035, -7.2964)
  line L631 (39.035, -7.2964) -> (38.9874, -7.2131)
  line L632 (38.9874, -7.2131) -> (38.9493, -7.1396)
  line L633 (38.9493, -7.1396) -> (38.8968, -7.0209)
  line L634 (38.8968, -7.0209) -> (38.8646, -6.9242)
  line L635 (38.8646, -6.9242) -> (38.8557, -6.8676)
  line L636 (38.8557, -6.8676) -> (38.832, -6.754)
  line L637 (38.832, -6.754) -> (38.8018, -6.6546)
  line L638 (38.8018, -6.6546) -> (38.7661, -6.5696)
  line L639 (38.7661, -6.5696) -> (38.7262, -6.4993)
  line L640 (38.7262, -6.4993) -> (38.6831, -6.4439)
  line L641 (38.6831, -6.4439) -> (38.6381, -6.4035)
  line L642 (38.6381, -6.4035) -> (38.6152, -6.3889)
  line L643 (38.6152, -6.3889) -> (38.5923, -6.3781)
  line L644 (38.5923, -6.3781) -> (38.5696, -6.3711)
  line L645 (38.5696, -6.3711) -> (38.547, -6.3678)
  line L646 (38.547, -6.3678) -> (38.5194, -6.3689)
  line L647 (38.5194, -6.3689) -> (38.2578, -6.4054)
  line L648 (38.2578, -6.4054) -> (38.1742, -6.4147)
  line L649 (38.1742, -6.4147) -> (38.0905, -6.4229)
  line L650 (38.0905, -6.4229) -> (37.8271, -6.4417)
  line L651 (37.8271, -6.4417) -> (37.7998, -6.4463)
  line L652 (37.7998, -6.4463) -> (37.7784, -6.4543)
  line L653 (37.7784, -6.4543) -> (37.7576, -6.4659)
  line L654 (37.7576, -6.4659) -> (37.7375, -6.4812)
  line L655 (37.7375, -6.4812) -> (37.7181, -6.5002)
  line L656 (37.7181, -6.5002) -> (37.6825, -6.5491)
  line L657 (37.6825, -6.5491) -> (37.6519, -6.6122)
  line L658 (37.6519, -6.6122) -> (37.6274, -6.6893)
  line L659 (37.6274, -6.6893) -> (37.6102, -6.7798)
  line L660 (37.6102, -6.7798) -> (37.6013, -6.8834)
  line L661 (37.6013, -6.8834) -> (37.6018, -6.9994)
  line L662 (37.6018, -6.9994) -> (37.6048, -7.0566)
  line L663 (37.6048, -7.0566) -> (37.5935, -7.1579)
  line L664 (37.5935, -7.1579) -> (37.5667, -7.2849)
  line L665 (37.5667, -7.2849) -> (37.5448, -7.3648)
  line L666 (37.5448, -7.3648) -> (37.5155, -7.4561)
  line L667 (37.5155, -7.4561) -> (37.4783, -7.5575)
  line L668 (37.4783, -7.5575) -> (37.4323, -7.6684)
  line L669 (37.4323, -7.6684) -> (37.3751, -7.7911)
  line L670 (37.3751, -7.7911) -> (37.309, -7.919)
  line L671 (37.309, -7.919) -> (37.2307, -8.0558)
  line L672 (37.2307, -8.0558) -> (37.1404, -8.1995)
  line L673 (37.1404, -8.1995) -> (37.0368, -8.3499)
  line L674 (37.0368, -8.3499) -> (36.9384, -8.4814)
  arc A16 (36.286, -8.4128) -> (36.9384, -8.4814) centre (37.5, 0) ccw
  line L675 (36.286, -8.4128) -> (36.217, -8.2637)
  line L676 (36.217, -8.2637) -> (36.147, -8.0951)
  line L677 (36.147, -8.0951) -> (36.0885, -7.9358)
  line L678 (36.0885, -7.9358) -> (36.0404, -7.7856)
  line L679 (36.0404, -7.7856) -> (36.0023, -7.6468)
  line L680 (36.0023, -7.6468) -> (35.9719, -7.5149)
  line L681 (35.9719, -7.5149) -> (35.9499, -7.3968)
  line L682 (35.9499, -7.3968) -> (35.9346, -7.2899)
  line L683 (35.9346, -7.2899) -> (35.925, -7.1945)
  line L684 (35.925, -7.1945) -> (35.9201, -7.1118)
  line L685 (35.9201, -7.1118) -> (35.9204, -6.982)
  line L686 (35.9204, -6.982) -> (35.9303, -6.8806)
  line L687 (35.9303, -6.8806) -> (35.9451, -6.8253)
  line L688 (35.9451, -6.8253) -> (35.9698, -6.7119)
  line L689 (35.9698, -6.7119) -> (35.9826, -6.6088)
  line L690 (35.9826, -6.6088) -> (35.9846, -6.5166)
  line L691 (35.9846, -6.5166) -> (35.9767, -6.4361)
  line L692 (35.9767, -6.4361) -> (35.9599, -6.368)
  line L693 (35.9599, -6.368) -> (35.9352, -6.3128)
  line L694 (35.9352, -6.3128) -> (35.9202, -6.2902)
  line L695 (35.9202, -6.2902) -> (35.9037, -6.271)
  line L696 (35.9037, -6.271) -> (35.8857, -6.2553)
  line L697 (35.8857, -6.2553) -> (35.8665, -6.2431)
  line L698 (35.8665, -6.2431) -> (35.8408, -6.2329)
  line L699 (35.8408, -6.2329) -> (35.587, -6.1598)
  line L700 (35.587, -6.1598) -> (35.5068, -6.1343)
  line L701 (35.5068, -6.1343) -> (35.427, -6.1078)
  line L702 (35.427, -6.1078) -> (35.1787, -6.0178)
  line L703 (35.1787, -6.0178) -> (35.1519, -6.011)
  line L704 (35.1519, -6.011) -> (35.1292, -6.0095)
  line L705 (35.1292, -6.0095) -> (35.1054, -6.0117)
  line L706 (35.1054, -6.0117) -> (35.0808, -6.0175)
  line L707 (35.0808, -6.0175) -> (35.0554, -6.0269)
  line L708 (35.0554, -6.0269) -> (35.003, -6.0571)
  line L709 (35.003, -6.0571) -> (34.9493, -6.1023)
  line L710 (34.9493, -6.1023) -> (34.8956, -6.1628)
  line L711 (34.8956, -6.1628) -> (34.8431, -6.2385)
  line L712 (34.8431, -6.2385) -> (34.7928, -6.3295)
  line L713 (34.7928, -6.3295) -> (34.7461, -6.4357)
  line L714 (34.7461, -6.4357) -> (34.7256, -6.4892)
  line L715 (34.7256, -6.4892) -> (34.674, -6.5771)
  line L716 (34.674, -6.5771) -> (34.5979, -6.6822)
  line L717 (34.5979, -6.6822) -> (34.5454, -6.7463)
  line L718 (34.5454, -6.7463) -> (34.4815, -6.8178)
  line L719 (34.4815, -6.8178) -> (34.4063, -6.8953)
  line L720 (34.4063, -6.8953) -> (34.3191, -6.9779)
  line L721 (34.3191, -6.9779) -> (34.217, -7.0668)
  line L722 (34.217, -7.0668) -> (34.1045, -7.1566)
  line L723 (34.1045, -7.1566) -> (33.9774, -7.2498)
  line L724 (33.9774, -7.2498) -> (33.8364, -7.3444)
  line L725 (33.8364, -7.3444) -> (33.6807, -7.4396)
  line L726 (33.6807, -7.4396) -> (33.5372, -7.5197)
  arc A17 (32.9691, -7.1917) -> (33.5372, -7.5197) centre (37.5, 0) ccw
  line L727 (32.9691, -7.1917) -> (32.9668, -7.0275)
  line L728 (32.9668, -7.0275) -> (32.9714, -6.8449)
  line L729 (32.9714, -6.8449) -> (32.9828, -6.6756)
  line L730 (32.9828, -6.6756) -> (32.9999, -6.5189)
  line L731 (32.9999, -6.5189) -> (33.0215, -6.3765)
  line L732 (33.0215, -6.3765) -> (33.0474, -6.2437)
  line L733 (33.0474, -6.2437) -> (33.0754, -6.1269)
  line L734 (33.0754, -6.1269) -> (33.1049, -6.0229)
  line L735 (33.1049, -6.0229) -> (33.1349, -5.9319)
  line L736 (33.1349, -5.9319) -> (33.1641, -5.8544)
  line L737 (33.1641, -5.8544) -> (33.2171, -5.7359)
  line L738 (33.2171, -5.7359) -> (33.2674, -5.6473)
  line L739 (33.2674, -5.6473) -> (33.3035, -5.6028)
  line L740 (33.3035, -5.6028) -> (33.3721, -5.5092)
  line L741 (33.3721, -5.5092) -> (33.4258, -5.4202)
  line L742 (33.4258, -5.4202) -> (33.4651, -5.3368)
  line L743 (33.4651, -5.3368) -> (33.4906, -5.2601)
  line L744 (33.4906, -5.2601) -> (33.5029, -5.191)
  line L745 (33.5029, -5.191) -> (33.5028, -5.1306)
  line L746 (33.5028, -5.1306) -> (33.4983, -5.1038)
  line L747 (33.4983, -5.1038) -> (33.491, -5.0796)
  line L748 (33.491, -5.0796) -> (33.481, -5.0579)
  line L749 (33.481, -5.0579) -> (33.4684, -5.039)
  line L750 (33.4684, -5.039) -> (33.4491, -5.0192)
  line L751 (33.4491, -5.0192) -> (33.2469, -4.8492)
  line L752 (33.2469, -4.8492) -> (33.1841, -4.7933)
  line L753 (33.1841, -4.7933) -> (33.122, -4.7366)
  line L754 (33.122, -4.7366) -> (32.9317, -4.5534)
  line L755 (32.9317, -4.5534) -> (32.9101, -4.5363)
  line L756 (32.9101, -4.5363) -> (32.8899, -4.5257)
  line L757 (32.8899, -4.5257) -> (32.8673, -4.518)
  line L758 (32.8673, -4.518) -> (32.8424, -4.5132)
  line L759 (32.8424, -4.5132) -> (32.8154, -4.5116)
  line L760 (32.8154, -4.5116) -> (32.7552, -4.5178)
  line L761 (32.7552, -4.5178) -> (32.6878, -4.5373)
  line L762 (32.6878, -4.5373) -> (32.6142, -4.5707)
  line L763 (32.6142, -4.5707) -> (32.5353, -4.6185)
  line L764 (32.5353, -4.6185) -> (32.4524, -4.6812)
  line L765 (32.4524, -4.6812) -> (32.3666, -4.7592)
  line L766 (32.3666, -4.7592) -> (32.3261, -4.7997)
  line L767 (32.3261, -4.7997) -> (32.2432, -4.859)
  line L768 (32.2432, -4.859) -> (32.1309, -4.9241)
  line L769 (32.1309, -4.9241) -> (32.0569, -4.9613)
  line L770 (32.0569, -4.9613) -> (31.9695, -5.0006)
  line L771 (31.9695, -5.0006) -> (31.8692, -5.0408)
  line L772 (31.8692, -5.0408) -> (31.756, -5.0808)
  line L773 (31.756, -5.0808) -> (31.6265, -5.1205)
  line L774 (31.6265, -5.1205) -> (31.4872, -5.1568)
  line L775 (31.4872, -5.1568) -> (31.3332, -5.1903)
  line L776 (31.3332, -5.1903) -> (31.1659, -5.2193)
  line L777 (31.1659, -5.2193) -> (30.9849, -5.243)
  line L778 (30.9849, -5.243) -> (30.8213, -5.2578)
  arc A18 (30.4357, -4.7271) -> (30.8213, -5.2578) centre (37.5, 0) ccw
  line L779 (30.4357, -4.7271) -> (30.5004, -4.5761)
  line L780 (30.676, 2.741) -> (30.453, 2.6211)
  line L781 (30.453, 2.6211) -> (30.2376, 2.5111)
  line L782 (30.2376, 2.5111) -> (30.0323, 2.4116)
  line L783 (30.0323, 2.4116) -> (29.8355, 2.3213)
  line L784 (29.8355, 2.3213) -> (29.6473, 2.2396)
  line L785 (29.6473, 2.2396) -> (29.4705, 2.1673)
  line L786 (29.4705, 2.1673) -> (29.3033, 2.1029)
  line L787 (29.3033, 2.1029) -> (28.9724, 1.9849)
  line L788 (28.9724, 1.9849) -> (28.931, 1.9629)
  line L789 (28.931, 1.9629) -> (28.9033, 1.9404)
  line L790 (28.9033, 1.9404) -> (28.8892, 1.9178)
  line L791 (28.8892, 1.9178) -> (28.8876, 1.9012)
  line L792 (28.8876, 1.9012) -> (28.9103, 1.5151)
  line L793 (28.9103, 1.5151) -> (28.9281, 1.1288)
  line L794 (28.9281, 1.1288) -> (28.9314, 1.1124)
  line L795 (28.9314, 1.1124) -> (28.9478, 1.0915)
  line L796 (28.9478, 1.0915) -> (28.9777, 1.0719)
  line L797 (28.9777, 1.0719) -> (29.0211, 1.0544)
  line L798 (29.0211, 1.0544) -> (29.3626, 0.9717)
  line L799 (29.3626, 0.9717) -> (29.5356, 0.9251)
  line L800 (29.5356, 0.9251) -> (29.719, 0.8717)
  line L801 (29.719, 0.8717) -> (29.9147, 0.8101)
  line L802 (29.9147, 0.8101) -> (30.1199, 0.7408)
  line L803 (30.1199, 0.7408) -> (30.3344, 0.6634)
  line L804 (30.3344, 0.6634) -> (30.5601, 0.5765)
  line L805 (30.5601, 0.5765) -> (30.7945, 0.4805)
  line L806 (30.7945, 0.4805) -> (30.9975, 0.3928)
  arc A19 (30.9975, -0.3928) -> (30.9975, 0.3928) centre (0, 0) ccw
  line L807 (30.9975, -0.3928) -> (30.7945, -0.4805)
  line L808 (30.7945, -0.4805) -> (30.5601, -0.5765)
  line L809 (30.5601, -0.5765) -> (30.3344, -0.6634)
  line L810 (30.3344, -0.6634) -> (30.1199, -0.7408)
  line L811 (30.1199, -0.7408) -> (29.9147, -0.8101)
  line L812 (29.9147, -0.8101) -> (29.719, -0.8717)
  line L813 (29.719, -0.8717) -> (29.5356, -0.9251)
  line L814 (29.5356, -0.9251) -> (29.3626, -0.9717)
  line L815 (29.3626, -0.9717) -> (29.0211, -1.0544)
  line L816 (29.0211, -1.0544) -> (28.9777, -1.0719)
  line L817 (28.9777, -1.0719) -> (28.9478, -1.0915)
  line L818 (28.9478, -1.0915) -> (28.9314, -1.1124)
  line L819 (28.9314, -1.1124) -> (28.9281, -1.1288)
  line L820 (28.9281, -1.1288) -> (28.9103, -1.5151)
  line L821 (28.9103, -1.5151) -> (28.8876, -1.9012)
  line L822 (28.8876, -1.9012) -> (28.8892, -1.9178)
  line L823 (28.8892, -1.9178) -> (28.9033, -1.9404)
  line L824 (28.9033, -1.9404) -> (28.931, -1.9629)
  line L825 (28.931, -1.9629) -> (28.9724, -1.9849)
  line L826 (28.9724, -1.9849) -> (29.3033, -2.1029)
  line L827 (29.3033, -2.1029) -> (29.4705, -2.1673)
  line L828 (29.4705, -2.1673) -> (29.6473, -2.2396)
  line L829 (29.6473, -2.2396) -> (29.8355, -2.3213)
  line L830 (29.8355, -2.3213) -> (30.0323, -2.4116)
  line L831 (30.0323, -2.4116) -> (30.2376, -2.5111)
  line L832 (30.2376, -2.5111) -> (30.453, -2.6211)
  line L833 (30.453, -2.6211) -> (30.676, -2.741)
  line L834 (30.676, -2.741) -> (30.8688, -2.8495)
  arc A20 (30.7866, -3.6308) -> (30.8688, -2.8495) centre (0, 0) ccw
  line L835 (30.7866, -3.6308) -> (30.5755, -3.6968)
  line L836 (30.5755, -3.6968) -> (30.3325, -3.7677)
  line L837 (30.3325, -3.7677) -> (30.0989, -3.8305)
  line L838 (30.0989, -3.8305) -> (29.8774, -3.8852)
  line L839 (29.8774, -3.8852) -> (29.6661, -3.9326)
  line L840 (29.6661, -3.9326) -> (29.465, -3.9734)
  line L841 (29.465, -3.9734) -> (29.2771, -4.0074)
  line L842 (29.2771, -4.0074) -> (29.1001, -4.0356)
  line L843 (29.1001, -4.0356) -> (28.7519, -4.0822)
  line L844 (28.7519, -4.0822) -> (28.7069, -4.0951)
  line L845 (28.7069, -4.0951) -> (28.6751, -4.1114)
  line L846 (28.6751, -4.1114) -> (28.6567, -4.1305)
  line L847 (28.6567, -4.1305) -> (28.6516, -4.1464)
  line L848 (28.6516, -4.1464) -> (28.5936, -4.5288)
  line L849 (28.5936, -4.5288) -> (28.5306, -4.9104)
  line L850 (28.5306, -4.9104) -> (28.5305, -4.927)
  line L851 (28.5305, -4.927) -> (28.5421, -4.951)
  line L852 (28.5421, -4.951) -> (28.5674, -4.9763)
  line L853 (28.5674, -4.9763) -> (28.6062, -5.0025)
  line L854 (28.6062, -5.0025) -> (28.9229, -5.1544)
  line L855 (28.9229, -5.1544) -> (29.0826, -5.2359)
  line L856 (29.0826, -5.2359) -> (29.2508, -5.3263)
  line L857 (29.2508, -5.3263) -> (29.4294, -5.4272)
  line L858 (29.4294, -5.4272) -> (29.6157, -5.5376)
  line L859 (29.6157, -5.5376) -> (29.8094, -5.658)
  line L860 (29.8094, -5.658) -> (30.0122, -5.79)
  line L861 (30.0122, -5.79) -> (30.2214, -5.9325)
  line L862 (30.2214, -5.9325) -> (30.4018, -6.0605)
  arc A21 (30.2385, -6.829) -> (30.4018, -6.0605) centre (0, 0) ccw
  line L863 (30.2385, -6.829) -> (30.0216, -6.8726)
  line L864 (30.0216, -6.8726) -> (29.7725, -6.9177)
  line L865 (29.7725, -6.9177) -> (29.5336, -6.9557)
  line L866 (29.5336, -6.9557) -> (29.3077, -6.9869)
  line L867 (29.3077, -6.9869) -> (29.0926, -7.012)
  line L868 (29.0926, -7.012) -> (28.8883, -7.0315)
  line L869 (28.8883, -7.0315) -> (28.6979, -7.0457)
  line L870 (28.6979, -7.0457) -> (28.5189, -7.0553)
  line L871 (28.5189, -7.0553) -> (28.1677, -7.0652)
  line L872 (28.1677, -7.0652) -> (28.1216, -7.0733)
  line L873 (28.1216, -7.0733) -> (28.0883, -7.0862)
  line L874 (28.0883, -7.0862) -> (28.0679, -7.1033)
  line L875 (28.0679, -7.1033) -> (28.0612, -7.1186)
  line L876 (28.0612, -7.1186) -> (27.9636, -7.4928)
  line L877 (27.9636, -7.4928) -> (27.861, -7.8657)
  line L878 (27.861, -7.8657) -> (27.8592, -7.8823)
  line L879 (27.8592, -7.8823) -> (27.8683, -7.9073)
  line L880 (27.8683, -7.9073) -> (27.8907, -7.9351)
  line L881 (27.8907, -7.9351) -> (27.9266, -7.9652)
  line L882 (27.9266, -7.9652) -> (28.2257, -8.1494)
  line L883 (28.2257, -8.1494) -> (28.3759, -8.2472)
  line L884 (28.3759, -8.2472) -> (28.5338, -8.3547)
  line L885 (28.5338, -8.3547) -> (28.7009, -8.4737)
  line L886 (28.7009, -8.4737) -> (28.8746, -8.603)
  line L887 (28.8746, -8.603) -> (29.0547, -8.7429)
  line L888 (29.0547, -8.7429) -> (29.2425, -8.8954)
  line L889 (29.2425, -8.8954) -> (29.4358, -9.059)
  line L890 (29.4358, -9.059) -> (29.6018, -9.2052)
  arc A22 (29.359, -9.9523) -> (29.6018, -9.2052) centre (0, 0) ccw
  line L891 (29.359, -9.9523) -> (29.1388, -9.973)
  line L892 (29.1388, -9.973) -> (28.8863, -9.9918)
  line L893 (28.8863, -9.9918) -> (28.6447, -10.0047)
  line L894 (28.6447, -10.0047) -> (28.4168, -10.0121)
  line L895 (28.4168, -10.0121) -> (28.2002, -10.0146)
  line L896 (28.2002, -10.0146) -> (27.995, -10.0127)
  line L897 (27.995, -10.0127) -> (27.8042, -10.0069)
  line L898 (27.8042, -10.0069) -> (27.6252, -9.9977)
  line L899 (27.6252, -9.9977) -> (27.2749, -9.9708)
  line L900 (27.2749, -9.9708) -> (27.2282, -9.9741)
  line L901 (27.2282, -9.9741) -> (27.1937, -9.9834)
  line L902 (27.1937, -9.9834) -> (27.1717, -9.9983)
  line L903 (27.1717, -9.9983) -> (27.1634, -10.0128)
  line L904 (27.1634, -10.0128) -> (27.0272, -10.3748)
  line L905 (27.0272, -10.3748) -> (26.8862, -10.7349)
  line L906 (26.8862, -10.7349) -> (26.8826, -10.7512)
  line L907 (26.8826, -10.7512) -> (26.8891, -10.777)
  line L908 (26.8891, -10.777) -> (26.9085, -10.807)
  line L909 (26.9085, -10.807) -> (26.941, -10.8407)
  line L910 (26.941, -10.8407) -> (27.2193, -11.0551)
  line L911 (27.2193, -11.0551) -> (27.3584, -11.1681)
  line L912 (27.3584, -11.1681) -> (27.5042, -11.2915)
  line L913 (27.5042, -11.2915) -> (27.6579, -11.4273)
  line L914 (27.6579, -11.4273) -> (27.8172, -11.5741)
  line L915 (27.8172, -11.5741) -> (27.9817, -11.7321)
  line L916 (27.9817, -11.7321) -> (28.1525, -11.9033)
  line L917 (28.1525, -11.9033) -> (28.3276, -12.0862)
  line L918 (28.3276, -12.0862) -> (28.4774, -12.249)
  arc A23 (28.1579, -12.9667) -> (28.4774, -12.249) centre (0, 0) ccw
  line L919 (28.1579, -12.9667) -> (27.9367, -12.9642)
  line L920 (27.9367, -12.9642) -> (27.6836, -12.9565)
  line L921 (27.6836, -12.9565) -> (27.442, -12.9441)
  line L922 (27.442, -12.9441) -> (27.2145, -12.9276)
  line L923 (27.2145, -12.9276) -> (26.9989, -12.9075)
  line L924 (26.9989, -12.9075) -> (26.7951, -12.8841)
  line L925 (26.7951, -12.8841) -> (26.6059, -12.8584)